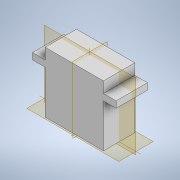
# Autodesk Inventor part: Motortest
Saved by Autodesk Inventor 2021 (Build 250183000, 183)
## iProperties
Created: 2022-11-29
Part Number: Motortest
Material: Generisch
Document SubType Name: Modeling
Designer: Elian
Density: 1 g/cm^3
Appearance: Vorgabe
Author: Elian
Autodesk Inventor part; units mm, degrees
sketch "Skizze1" plane through (0, 0, 0) normal (0, 0, 1) x (1, 0, 0)
  line L0 (-11.25, 0) -> (11.25, 0)
  line L1 (11.25, 0) -> (11.25, 16.7)
  line L2 (11.25, 16.7) -> (-11.25, 16.7)
  line L3 (-11.25, 16.7) -> (-11.25, 0)
  line L4 (0, -4.68) -> (0, 28.08) projected
  line L5 (-11.25, 16.7) -> (-16.15, 16.7)
  line L6 (-16.15, 16.7) -> (-16.15, 19.2)
  line L7 (-16.15, 19.2) -> (-11.25, 19.2)
  line L8 (-11.25, 19.2) -> (-11.25, 23.4)
  line L9 (-11.25, 23.4) -> (0, 23.4)
  line L10 (11.25, 16.7) -> (16.15, 16.7)
  line L11 (16.15, 16.7) -> (16.15, 19.2)
  line L12 (16.15, 19.2) -> (11.25, 19.2)
  line L13 (11.25, 19.2) -> (11.25, 23.4)
  line L14 (11.25, 23.4) -> (0, 23.4)
  point P0 (0, 0)
  dimension "d0" = 22.5
  dimension "d1" = 16.7
  dimension "d2" = 4.9
  dimension "d3" = 2.5
  dimension "d4" = 4.2
  dimension "d5" = 22.5
  constraints: 28 end point, 4 perpendicular, 4 symmetric about line, 3 horizontal, 2 parallel, 1 point on line, 1 other
  measures "d0" distance of L0.start L0.end
  measures "d1" distance of L0.end L1.end
  measures "d2" distance of L2.end L5.end
  measures "d3" distance of L5.end L6.end
  measures "d4" distance of L7.end L8.end
  measures "d5" distance of L8.end L14.start
extrude "Extrusion1" add sketch "Skizze1" along normal mid plane 12.1
